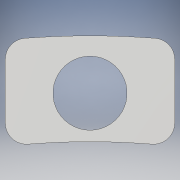
# Autodesk Inventor part: Reverse Gear Link Block
Saved by Autodesk Inventor 2017 (Build 210142000, 142)
## iProperties
Created: 2018-11-11
Part Number: Reverse Gear Link Block
Material: PVC-Piping
Document SubType Name: Modeling
Designer: Arman Grewal
Density: 1.4 g/cm^3
Appearance: Smooth - White
Author: Arman Grewal
Autodesk Inventor part; units mm, degrees
ref_plane "YZ Plane" through (0, 0, 0) normal (1, 0, 0) x (0, 1, 0)
ref_plane "XZ Plane" through (0, 0, 0) normal (0, 1, 0) x (-1, 0, 0)
ref_plane "XY Plane" through (0, 0, 0) normal (0, 0, 1) x (1, 0, 0)
sketch "Sketch1" plane through (0, 0, 0) normal (1, 0, 0) x (0, 1, 0)
  circle A0 centre (0, 0) radius 43.75 construction
  circle A1 centre (0, 0) radius 38.75 construction
  line L0 (48.236, 0) -> (48.236, 4) construction
  line L1 (48.236, 0) -> (48.236, -4) construction
  arc A2 (43.5668, -4) -> (43.5668, 4) centre (0, 0) ccw construction
  arc A3 (38.543, -4) -> (38.543, 4) centre (0, 0) ccw construction
  line L2 (43.5668, 4) -> (38.543, 4)
  line L3 (38.543, -4) -> (43.5668, -4)
  arc A4 (38.543, -4) -> (38.543, 4) centre (3.2648, 0) ccw
  arc A5 (43.5668, -4) -> (43.5668, 4) centre (3.2648, 0) ccw
  line L4 (38.769, 0) -> (43.7648, 0) construction
  line L5 (41.0549, 4) -> (41.0549, -4) construction
  circle A6 centre (41.0549, 0) radius 1.75 construction
  circle A7 centre (41.0549, 0) radius 1.75
  dimension "d0" = 87.5
  dimension "d1" = 77.5
  dimension "d2" = 4
  dimension "d3" = 4
  dimension "d4" = 3.5
  dimension "d5" = 3.5
  dimension "d6" = 40.5
  dimension "d7" = 7.1811
  dimension "d8" = 4
  dimension "d9" = 4
  constraints: 14 point on circle, 12 end point, 8 centre point, 3 coincident, 3 concentric, 3 midpoint, 2 vertical, 1 horizontal, 1 parallel
  measures "d0" diameter of A0
  measures "d1" diameter of A1
  measures "d2" distance of L0.start L0.end
  measures "d3" distance of L0.start L1.end
  measures "d4" diameter of A6
  measures "d5" diameter of A7
  measures "d6" radius of A5
  measures "d7" distance between parallel lines of L0 L5
  measures "d8" distance between parallel lines of L2 L4
  measures "d9" distance from line of L0.end L4
extrude "Extrusion2" add sketch "Sketch1" along normal blind 3
fillet "Fillet2" radius 1 4 edges at (1.5, 43.5668, -4) (1.5, 43.5668, 4) (1.5, 38.543, 4) (1.5, 38.543, -4)
body "Solid2"
